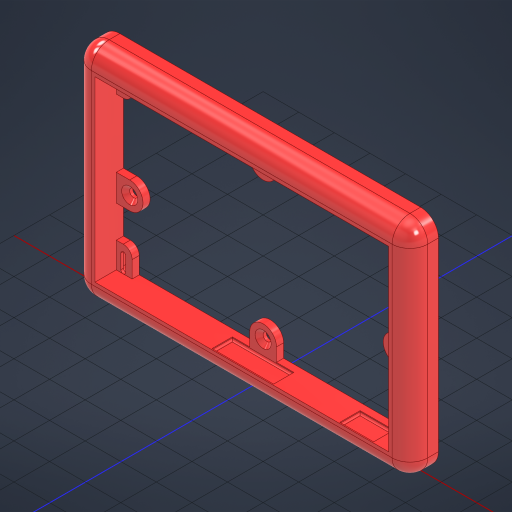
# Autodesk Inventor part: Display_Bevel
Saved by Autodesk Inventor 2023.2 (Build 272271030, 271C)
## iProperties
Created: 2023-04-02
Part Number: Display_Bevel
Material: Generisch
Document SubType Name: Modeling
Designer: Stefan
Mass: 99.9269 g
Surface Area: 326.591 cm^2
Volume: 99.9269 cm^3
Density: 1 g/cm^3
Appearance: Hellrot
Author: Stefan
Autodesk Inventor part; units mm, degrees
ref_plane "YZ Plane" through (0, 0, 0) normal (1, 0, 0) x (0, 1, 0)
ref_plane "XZ Plane" through (0, 0, 0) normal (0, 1, 0) x (-1, 0, 0)
ref_plane "XY Plane" through (0, 0, 0) normal (0, 0, 1) x (1, 0, 0)
sketch "Skizze1" plane through (0, 0, 0) normal (0, 0, 1) x (1, 0, 0)
  line L0 (-82.5, -50) -> (82.5, -50)
  line L1 (82.5, -50) -> (82.5, 50)
  line L2 (82.5, 50) -> (-82.5, 50)
  line L3 (-82.5, 50) -> (-82.5, -50)
  line L4 (-82.5, -50) -> (82.5, 50) construction
  line L5 (82.5, -50) -> (-82.5, 50) construction
  line L6 (-94.5, -62) -> (94.5, -62)
  line L7 (94.5, -62) -> (94.5, 62)
  line L8 (94.5, 62) -> (-94.5, 62)
  line L9 (-94.5, 62) -> (-94.5, -62)
  line L10 (-78.6, -44.6) -> (78.6, -44.6) construction
  line L11 (78.6, -44.6) -> (78.6, 44.6) construction
  line L12 (78.6, 44.6) -> (-78.6, 44.6) construction
  line L13 (-78.6, 44.6) -> (-78.6, -44.6) construction
  line L14 (73.5, -50) -> (54.5, -50)
  line L15 (54.5, -50) -> (54.5, -51.5)
  line L16 (54.5, -51.5) -> (73.5, -51.5)
  line L17 (73.5, -51.5) -> (73.5, -50)
  line L18 (-78.6, -40.55) -> (-78.6, -48.65) construction
  line L19 (-79.95, -40.55) -> (-79.95, -48.65)
  line L20 (-77.25, -48.65) -> (-77.25, -40.55)
  arc A0 (-77.25, -40.55) -> (-79.95, -40.55) centre (-78.6, -40.55) ccw
  arc A1 (-79.95, -48.65) -> (-77.25, -48.65) centre (-78.6, -48.65) ccw
  line L21 (78.6, -40.55) -> (78.6, -48.65) construction
  line L22 (77.25, -40.55) -> (77.25, -48.65)
  line L23 (79.95, -48.65) -> (79.95, -40.55)
  arc A2 (79.95, -40.55) -> (77.25, -40.55) centre (78.6, -40.55) ccw
  arc A3 (77.25, -48.65) -> (79.95, -48.65) centre (78.6, -48.65) ccw
  line L24 (-78.6, 48.65) -> (-78.6, 40.55) construction
  line L25 (-79.95, 48.65) -> (-79.95, 40.55)
  line L26 (-77.25, 40.55) -> (-77.25, 48.65)
  arc A4 (-77.25, 48.65) -> (-79.95, 48.65) centre (-78.6, 48.65) ccw
  arc A5 (-79.95, 40.55) -> (-77.25, 40.55) centre (-78.6, 40.55) ccw
  line L27 (78.6, 40.55) -> (78.6, 48.65) construction
  line L28 (79.95, 40.55) -> (79.95, 48.65)
  line L29 (77.25, 48.65) -> (77.25, 40.55)
  arc A6 (77.25, 40.55) -> (79.95, 40.55) centre (78.6, 40.55) ccw
  arc A7 (79.95, 48.65) -> (77.25, 48.65) centre (78.6, 48.65) ccw
  arc A8 (-78.6, 35.55) -> (-73.6, 40.55) centre (-78.6, 40.55) ccw
  line L30 (-78.6, 35.55) -> (-82.5, 35.55)
  line L31 (-73.6, 40.55) -> (-73.6, 50)
  arc A9 (73.6, 40.55) -> (78.6, 35.55) centre (78.6, 40.55) ccw
  arc A10 (-73.6, -40.55) -> (-78.6, -35.55) centre (-78.6, -40.55) ccw
  arc A11 (78.6, -35.55) -> (73.6, -40.55) centre (78.6, -40.55) ccw
  line L32 (-78.6, -35.55) -> (-82.5, -35.55)
  line L33 (-73.6, -40.55) -> (-73.6, -50)
  line L34 (73.6, -40.55) -> (73.6, -50)
  line L35 (78.6, -35.55) -> (82.5, -35.55)
  line L36 (73.6, 40.55) -> (73.6, 50)
  line L37 (78.6, 35.55) -> (82.5, 35.55)
  line L38 (-7.5, 50) -> (7.5, 50)
  line L39 (7.5, 50) -> (7.5, 42.5)
  line L40 (7.5, 42.5) -> (-7.5, 42.5) construction
  line L41 (-7.5, 42.5) -> (-7.5, 50)
  line L42 (-82.5, -2.5) -> (-75, -2.5)
  line L43 (-75, -2.5) -> (-75, -17.5) construction
  line L44 (-75, -17.5) -> (-82.5, -17.5)
  line L45 (-82.5, -17.5) -> (-82.5, -2.5)
  line L46 (82.5, -2.5) -> (75, -2.5)
  line L47 (75, -2.5) -> (75, -17.5) construction
  line L48 (75, -17.5) -> (82.5, -17.5)
  line L49 (82.5, -17.5) -> (82.5, -2.5)
  line L50 (-7.5, -50) -> (7.5, -50)
  line L51 (7.5, -50) -> (7.5, -42.5)
  line L52 (7.5, -42.5) -> (-7.5, -42.5) construction
  line L53 (-7.5, -42.5) -> (-7.5, -50)
  arc A12 (-75, -17.5) -> (-75, -2.5) centre (-75, -10) ccw
  arc A13 (-7.5, 42.5) -> (7.5, 42.5) centre (0, 42.5) ccw
  arc A14 (75, -2.5) -> (75, -17.5) centre (75, -10) ccw
  arc A15 (7.5, -42.5) -> (-7.5, -42.5) centre (0, -42.5) ccw
  circle A16 centre (-75, -10) radius 2.25
  circle A17 centre (0, 42.5) radius 2.25
  circle A18 centre (0, -42.5) radius 2.25
  circle A19 centre (75, -10) radius 2.25
  circle A20 centre (0, 42.5) radius 4.5
  circle A21 centre (-75, -10) radius 4.5
  circle A22 centre (0, -42.5) radius 4.5
  circle A23 centre (75, -10) radius 4.5
  line L54 (-17.3, -50) -> (17.3, -50)
  line L55 (17.3, -50) -> (17.3, -51.5)
  line L56 (17.3, -51.5) -> (-17.3, -51.5)
  line L57 (-17.3, -51.5) -> (-17.3, -50)
  point P0 (0, 0)
  point P1 (-70.3, -50)
  point P2 (-82.5, -37.65)
  point P3 (82.5, -37.65)
  point P4 (70.3, -50)
  point P5 (-78.6, 0)
  point P6 (0, 44.6)
  point P7 (0, 50)
  point P8 (82.5, 0)
  point P9 (-82.5, 0)
  point P10 (0, 35)
  point P11 (-82.5, -10)
  point P12 (82.5, -10)
  point P13 (0, -50)
  dimension "d0" = 100
  dimension "d1" = 165
  dimension "d2" = 12
  dimension "d16" = 9
  dimension "d17" = 19
  dimension "d18" = 1.5
  dimension "d23" = 2.7
  dimension "d24" = 2.7
  dimension "d25" = 10.8
  dimension "d26" = 10.8
  dimension "d27" = 2.7
  dimension "d28" = 2.7
  dimension "d30" = 10.8
  dimension "d31" = 89.2
  dimension "d32" = 157.2
  dimension "d33" = 10.8
  dimension "d34" = 5
  dimension "d38" = 15
  dimension "d39" = 15
  dimension "d41" = 4.5
  dimension "d43" = 9
  dimension "d46" = 10
  dimension "d49" = 34.6
  constraints: 122 end point, 33 point on circle, 32 tangent, 24 centre point, 21 parallel, 20 point on line, 17 midpoint, 16 coincident, 14 perpendicular, 9 equal radius, 8 horizontal, 6 equal length, 2 horizontal alignment, 2 vertical, 1 collinear, 1 vertical alignment, 14 other
  measures "d0" distance of L2.end L3.end
  measures "d1" distance of L1.end L2.end
  measures "d2" distance between parallel lines of L2 L8
  measures "d16" distance between parallel lines of L17 L1
  measures "d17" distance of L15.end L16.end
  measures "d18" distance of L14.end L15.end
  measures "d23" distance between parallel lines of L19 L20
  measures "d24" distance between parallel lines of L23 L22
  measures "d27" distance between parallel lines of L26 L25
  measures "d28" distance between parallel lines of L28 L29
  measures "d31" distance between parallel lines of L10 L12
  measures "d32" distance between parallel lines of L11 L13
  measures "d34" radius of A8
  measures "d38" distance between parallel lines of L39 L41
  measures "d39" distance from line of point (0, 35) L38
  measures "d41" diameter of A17
  measures "d43" diameter of A20
  measures "d46" vertical distance of point (75, -10) point (0, 0)
  measures "d49" distance of L55.end L56.end
extrude "Extrusion1" add sketch "Skizze1" along normal blind 12 contours L0 L55 L56 L57 | L0 L17 L16 L15 | L9 L8 L7 L6
extrude "Extrusion2" add sketch "Skizze1" against normal blind 4 contours L0 L3 L32 A10 L33 | L0 L55 L56 L57 | L53 A15 L51 L0 | L3 L42 A12 L44 | L0 L17 L16 L15 | L3 L2 L31 A8 L30 | L34 A11 L35 L1 L0 | L2 L39 A13 L41 | L48 A14 L46 L1 | L2 L1 L37 A9 L36 | L9 L8 L7 L6 | A20 | A21 | A22 | A23
fillet "Rundung1" radius 10 4 edges at (-94.5, -62, 4) (94.5, -62, 4) (94.5, 62, 4) (-94.5, 62, 4)
fillet "Rundung2" radius 10 8 edges at (91.5711, 59.0711, 12) (0, 62, 12) (-91.5711, 59.0711, 12) (-94.5, 0, 12) (-91.5711, -59.0711, 12) (0, -62, 12) (91.5711, -59.0711, 12) (94.5, 0, 12)
extrude "Extrusion3" cut sketch "Skizze1" along normal blind 11.4 contours L0 L55 L56 L57 | L0 L17 L16 L15
fillet "Rundung3" radius 1 8 edges at (73.5, -51.5, 5.7) (64, -51.5, 11.4) (54.5, -51.5, 5.7) (64, -51.5, 0) (0, -51.5, 0) (17.3, -51.5, 5.7) (0, -51.5, 11.4) (-17.3, -51.5, 5.7)
sketch "Skizze2" plane through (0, 0, -4) normal (0, 0, -1) x (-1, 0, 0)
  arc A0 (94.5, 52) -> (84.5, 62) centre (84.5, 52) ccw projected
  line L0 (84.5, 62) -> (-84.5, 62) projected
  arc A1 (-84.5, 62) -> (-94.5, 52) centre (-84.5, 52) ccw projected
  line L1 (-94.5, 52) -> (-94.5, -52) projected
  arc A2 (-94.5, -52) -> (-84.5, -62) centre (-84.5, -52) ccw projected
  line L2 (-84.5, -62) -> (84.5, -62) projected
  arc A3 (84.5, -62) -> (94.5, -52) centre (84.5, -52) ccw projected
  line L3 (94.5, -52) -> (94.5, 52) projected
  line L4 (82.5, 35.55) -> (82.5, -2.5) projected
  line L5 (82.5, -35.55) -> (78.6, -35.55) projected
  arc A4 (78.6, -35.55) -> (73.6, -40.55) centre (78.6, -40.55) ccw projected
  line L6 (73.6, -40.55) -> (73.6, -50) projected
  line L7 (73.6, -50) -> (7.5, -50) projected
  line L8 (-73.6, -50) -> (-73.6, -40.55) projected
  arc A5 (-73.6, -40.55) -> (-78.6, -35.55) centre (-78.6, -40.55) ccw projected
  line L9 (-78.6, -35.55) -> (-82.5, -35.55) projected
  line L10 (-82.5, -35.55) -> (-82.5, -17.5) projected
  line L11 (-82.5, 35.55) -> (-78.6, 35.55) projected
  arc A6 (-78.6, 35.55) -> (-73.6, 40.55) centre (-78.6, 40.55) ccw projected
  line L12 (-73.6, 40.55) -> (-73.6, 50) projected
  line L13 (-73.6, 50) -> (-7.5, 50) projected
  line L14 (73.6, 50) -> (73.6, 40.55) projected
  arc A7 (73.6, 40.55) -> (78.6, 35.55) centre (78.6, 40.55) ccw projected
  line L15 (78.6, 35.55) -> (82.5, 35.55) projected
  arc A8 (77.25, -48.65) -> (79.95, -48.65) centre (78.6, -48.65) ccw projected
  line L16 (77.25, -48.65) -> (77.25, -40.55) projected
  arc A9 (79.95, -40.55) -> (77.25, -40.55) centre (78.6, -40.55) ccw projected
  line L17 (79.95, -40.55) -> (79.95, -48.65) projected
  arc A10 (-79.95, -48.65) -> (-77.25, -48.65) centre (-78.6, -48.65) ccw projected
  line L18 (-79.95, -48.65) -> (-79.95, -40.55) projected
  arc A11 (-77.25, -40.55) -> (-79.95, -40.55) centre (-78.6, -40.55) ccw projected
  line L19 (-77.25, -40.55) -> (-77.25, -48.65) projected
  arc A12 (-77.25, 48.65) -> (-79.95, 48.65) centre (-78.6, 48.65) ccw projected
  line L20 (-77.25, 48.65) -> (-77.25, 40.55) projected
  arc A13 (-79.95, 40.55) -> (-77.25, 40.55) centre (-78.6, 40.55) ccw projected
  line L21 (-79.95, 40.55) -> (-79.95, 48.65) projected
  arc A14 (79.95, 48.65) -> (77.25, 48.65) centre (78.6, 48.65) ccw projected
  line L22 (79.95, 48.65) -> (79.95, 40.55) projected
  arc A15 (77.25, 40.55) -> (79.95, 40.55) centre (78.6, 40.55) ccw projected
  line L23 (77.25, 40.55) -> (77.25, 48.65) projected
  line L24 (-78.6, 48.65) -> (-78.6, 40.55) construction
  line L25 (-81.1, 48.65) -> (-81.1, 40.55)
  line L26 (-76.1, 40.55) -> (-76.1, 48.65)
  arc A16 (-76.1, 48.65) -> (-81.1, 48.65) centre (-78.6, 48.65) ccw
  arc A17 (-81.1, 40.55) -> (-76.1, 40.55) centre (-78.6, 40.55) ccw
  line L27 (-78.6, -40.55) -> (-78.6, -48.65) construction
  line L28 (-81.1, -40.55) -> (-81.1, -48.65)
  line L29 (-76.1, -48.65) -> (-76.1, -40.55)
  arc A18 (-76.1, -40.55) -> (-81.1, -40.55) centre (-78.6, -40.55) ccw
  arc A19 (-81.1, -48.65) -> (-76.1, -48.65) centre (-78.6, -48.65) ccw
  line L30 (78.6, 48.65) -> (78.6, 40.55) construction
  line L31 (76.1, 48.65) -> (76.1, 40.55)
  line L32 (81.1, 40.55) -> (81.1, 48.65)
  arc A20 (81.1, 48.65) -> (76.1, 48.65) centre (78.6, 48.65) ccw
  arc A21 (76.1, 40.55) -> (81.1, 40.55) centre (78.6, 40.55) ccw
  line L33 (78.6, -40.55) -> (78.6, -48.65) construction
  line L34 (76.1, -40.55) -> (76.1, -48.65)
  line L35 (81.1, -48.65) -> (81.1, -40.55)
  arc A22 (81.1, -40.55) -> (76.1, -40.55) centre (78.6, -40.55) ccw
  arc A23 (76.1, -48.65) -> (81.1, -48.65) centre (78.6, -48.65) ccw
  line L36 (82.5, -17.5) -> (82.5, -35.55) projected
  line L37 (7.5, -50) -> (7.5, -42.5) projected
  arc A24 (7.5, -42.5) -> (-7.5, -42.5) centre (0, -42.5) ccw projected
  line L38 (-7.5, -42.5) -> (-7.5, -50) projected
  line L39 (-7.5, -50) -> (-73.6, -50) projected
  line L40 (-82.5, -17.5) -> (-75, -17.5) projected
  arc A25 (-75, -17.5) -> (-75, -2.5) centre (-75, -10) ccw projected
  line L41 (-75, -2.5) -> (-82.5, -2.5) projected
  line L42 (-82.5, -2.5) -> (-82.5, 35.55) projected
  line L43 (-7.5, 50) -> (-7.5, 42.5) projected
  arc A26 (-7.5, 42.5) -> (7.5, 42.5) centre (0, 42.5) ccw projected
  line L44 (7.5, 42.5) -> (7.5, 50) projected
  line L45 (7.5, 50) -> (73.6, 50) projected
  line L46 (82.5, -2.5) -> (75, -2.5) projected
  arc A27 (75, -2.5) -> (75, -17.5) centre (75, -10) ccw projected
  line L47 (75, -17.5) -> (82.5, -17.5) projected
  point P0 (0, 0)
  point P1 (-78.6, 44.6)
  point P2 (-78.6, -44.6)
  point P3 (78.6, 44.6)
  point P4 (78.6, -44.6)
  dimension "d50" = 5
  constraints: 32 end point, 16 point on circle, 16 tangent, 8 centre point, 7 parallel, 4 midpoint, 3 equal radius, 1 vertical
  measures "d50" distance between parallel lines of L25 L26
extrude "Extrusion4" cut sketch "Skizze2" against normal blind 2.5 contours A16 L26 A17 L25 | A18 L29 A19 L28 | A20 L32 A21 L31 | A22 L35 A23 L34
sketch "Skizze1 outline for Extrusion5" plane through (0, 0, 0) normal (0, 0, 1) x (1, 0, 0)
  circle A0 centre (0, -42.5) radius 4.5
  circle A1 centre (75, -10) radius 4.5
  circle A2 centre (0, 42.5) radius 4.5
  circle A3 centre (-75, -10) radius 4.5
extrude "Extrusion5" cut sketch "Skizze1 outline for Extrusion5" against normal blind 3 draft -45
equation "\"d23\" = d24"
equation "\"d26\" = d25"
equation "\"d27\" = d24"
equation "\"d28\" = d24"
equation "\"d30\" = d25"
equation "\"d33\" = d25"
